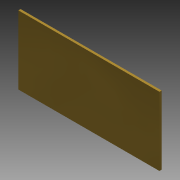
# Autodesk Inventor part: mid floater plate
Saved by Autodesk Inventor 2012 (Build 160160000, 160)
## iProperties
Created: 2013-05-10
Part Number: mid floater plate
Material: Gold
Document SubType Name: Modeling
Designer: Fabian
Mass: 257244 g
Surface Area: 14672.7 cm^2
Volume: 13328.7 cm^3
Density: 19.3 g/cm^3
Author: Fabian
Autodesk Inventor part; units mm, degrees
ref_plane "YZ Plane" through (0, 0, 0) normal (1, 0, 0) x (0, 1, 0)
ref_plane "XZ Plane" through (0, 0, 0) normal (0, 1, 0) x (-1, 0, 0)
ref_plane "XY Plane" through (0, 0, 0) normal (0, 0, 1) x (1, 0, 0)
sketch "Sketch1" plane through (0, 0, 0) normal (0, 0, 1) x (1, 0, 0)
  line L0 (-23.1469, 9.7902) -> (1176.8531, 9.7902)
  line L1 (1176.8531, 9.7902) -> (1176.8531, -573.2668)
  line L2 (1176.8531, -573.2668) -> (-23.1469, -573.2668)
  line L3 (-23.1469, -573.2668) -> (-23.1469, 9.7902)
  point P0 (0, 0)
  dimension "d0" = 1200
  dimension "d1" = 583.057
  constraints: 8 end point, 2 parallel, 1 horizontal, 1 perpendicular
  measures "d0" distance of L0.start L0.end
  measures "d1" distance of L2.end L0.start
extrude "Extrusion1" add sketch "Sketch1" along normal blind 19.05
body "Solid1"
